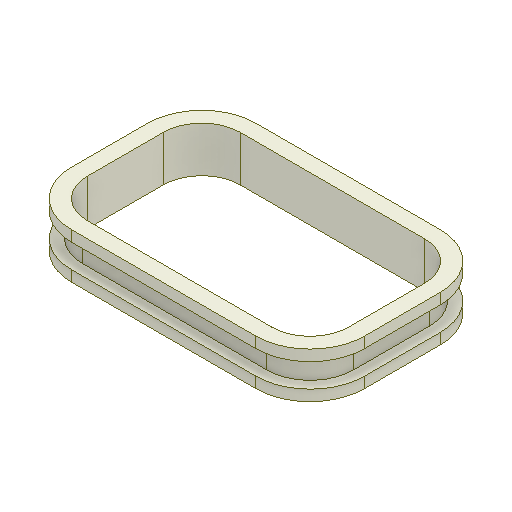
# Autodesk Inventor part: 3DP_TPU_Cable_Feed_Through_25mm
Saved by Autodesk Inventor 2026.1 (Build 301233000, 233)
## iProperties
Created: 2017-07-28
Part Number: 3DP_TPU_Cable_Feed_Through_25mm
Material: Ogólny
Document SubType Name: Modeling
Designer: Andrzej
Density: 1 g/cm^3
Appearance: Smooth - Ivory
Author: Andrzej
Autodesk Inventor part; units mm, degrees
ref_plane "YZ Plane" through (0, 0, 0) normal (1, 0, 0) x (0, 1, 0)
ref_plane "XZ Plane" through (0, 0, 0) normal (0, 1, 0) x (-1, 0, 0)
ref_plane "XY Plane" through (0, 0, 0) normal (0, 0, 1) x (1, 0, 0)
sketch "Szkic1" plane through (0, 0, 0) normal (0, 0, 1) x (1, 0, 0)
  line L0 (-2.3024, 6.9387) -> (14.6976, 6.9387)
  line L1 (18.6976, 2.9387) -> (18.6976, -4.0613)
  line L2 (14.6976, -8.0613) -> (-2.3024, -8.0613)
  line L3 (-6.3024, -4.0613) -> (-6.3024, 2.9387)
  arc A0 (-2.3024, 6.9387) -> (-6.3024, 2.9387) centre (-2.3024, 2.9387) ccw
  arc A1 (18.6976, 2.9387) -> (14.6976, 6.9387) centre (14.6976, 2.9387) ccw
  arc A2 (14.6976, -8.0613) -> (18.6976, -4.0613) centre (14.6976, -4.0613) ccw
  arc A3 (-6.3024, -4.0613) -> (-2.3024, -8.0613) centre (-2.3024, -4.0613) ccw
  line L4 (14.6976, 6.4887) -> (-2.3024, 6.4887)
  arc A4 (-2.3024, 6.4887) -> (-5.8524, 2.9387) centre (-2.3024, 2.9387) ccw
  line L5 (-5.8524, 2.9387) -> (-5.8524, -4.0613)
  arc A5 (-5.8524, -4.0613) -> (-2.3024, -7.6113) centre (-2.3024, -4.0613) ccw
  line L6 (-2.3024, -7.6113) -> (14.6976, -7.6113)
  arc A6 (14.6976, -7.6113) -> (18.2476, -4.0613) centre (14.6976, -4.0613) ccw
  line L7 (18.2476, -4.0613) -> (18.2476, 2.9387)
  arc A7 (18.2476, 2.9387) -> (14.6976, 6.4887) centre (14.6976, 2.9387) ccw
  point P0 (0, 0)
  point P1 (18.6976, -8.0613)
  point P2 (18.6976, 6.9387)
  point P3 (-6.3024, -8.0613)
  dimension "d0" = 25
  dimension "d1" = 15
  dimension "d2" = 4
  dimension "d3" = 0.45
  constraints: 16 end point, 16 point on circle, 8 centre point, 8 tangent, 6 point on line, 4 parallel, 3 equal radius, 2 perpendicular, 1 horizontal, 7 other
  measures "d0" distance of point (18.698, -8.061) point (-6.302, -8.061)
  measures "d1" distance of point (18.698, 6.939) point (18.698, -8.061)
  measures "d2" radius of A0
  measures "d3" distance between parallel lines of L0 L4
extrude "Wyciągnięcie proste1" add sketch "Szkic1" along normal blind 2.2
sketch "Szkic2" plane through (0, 0, 2.2) normal (0, 0, 1) x (1, 0, 0)
  arc A0 (18.2476, 2.9387) -> (14.6976, 6.4887) centre (14.6976, 2.9387) ccw projected
  line L0 (18.2476, 2.9387) -> (18.2476, -4.0613) projected
  arc A1 (14.6976, -7.6113) -> (18.2476, -4.0613) centre (14.6976, -4.0613) ccw projected
  line L1 (14.6976, -7.6113) -> (-2.3024, -7.6113) projected
  arc A2 (-5.8524, -4.0613) -> (-2.3024, -7.6113) centre (-2.3024, -4.0613) ccw projected
  line L2 (-5.8524, -4.0613) -> (-5.8524, 2.9387) projected
  arc A3 (-2.3024, 6.4887) -> (-5.8524, 2.9387) centre (-2.3024, 2.9387) ccw projected
  line L3 (-2.3024, 6.4887) -> (14.6976, 6.4887) projected
  line L4 (-6.3024, 2.9387) -> (-6.3024, -4.0613) projected
  arc A4 (-6.3024, -4.0613) -> (-2.3024, -8.0613) centre (-2.3024, -4.0613) ccw projected
  line L5 (-2.3024, -8.0613) -> (14.6976, -8.0613) projected
  arc A5 (14.6976, -8.0613) -> (18.6976, -4.0613) centre (14.6976, -4.0613) ccw projected
  line L6 (18.6976, -4.0613) -> (18.6976, 2.9387) projected
  arc A6 (18.6976, 2.9387) -> (14.6976, 6.9387) centre (14.6976, 2.9387) ccw projected
  line L7 (14.6976, 6.9387) -> (-2.3024, 6.9387) projected
  arc A7 (-2.3024, 6.9387) -> (-6.3024, 2.9387) centre (-2.3024, 2.9387) ccw projected
  line L8 (-7.3024, 2.9387) -> (-7.3024, -4.0613)
  arc A8 (-7.3024, -4.0613) -> (-2.3024, -9.0613) centre (-2.3024, -4.0613) ccw
  line L9 (-2.3024, -9.0613) -> (14.6976, -9.0613)
  arc A9 (14.6976, -9.0613) -> (19.6976, -4.0613) centre (14.6976, -4.0613) ccw
  line L10 (19.6976, -4.0613) -> (19.6976, 2.9387)
  arc A10 (19.6976, 2.9387) -> (14.6976, 7.9387) centre (14.6976, 2.9387) ccw
  line L11 (14.6976, 7.9387) -> (-2.3024, 7.9387)
  arc A11 (-2.3024, 7.9387) -> (-7.3024, 2.9387) centre (-2.3024, 2.9387) ccw
  point P0 (0, 0)
  dimension "d6" = 1
  constraints: 8 end point, 8 point on circle, 4 centre point, 7 other
  measures "d6" radial gap between concentric circles of A7 A11
extrude "Wyciągnięcie proste2" add sketch "Szkic2" along normal blind 1 contours A7 L7 A6 L6 A5 L5 A4 L4 | A11 L11 A10 L10 A9 L9 A8 L8
sketch "Szkic3" plane through (0, 0, 0) normal (0, 0, -1) x (-1, 0, 0)
  line L0 (7.3024, 2.9387) -> (7.3024, -4.0613) projected
  arc A0 (7.3024, 2.9387) -> (2.3024, 7.9387) centre (2.3024, 2.9387) ccw projected
  line L1 (-14.6976, 7.9387) -> (2.3024, 7.9387) projected
  arc A1 (-14.6976, 7.9387) -> (-19.6976, 2.9387) centre (-14.6976, 2.9387) ccw projected
  line L2 (-19.6976, -4.0613) -> (-19.6976, 2.9387) projected
  arc A2 (-19.6976, -4.0613) -> (-14.6976, -9.0613) centre (-14.6976, -4.0613) ccw projected
  line L3 (2.3024, -9.0613) -> (-14.6976, -9.0613) projected
  arc A3 (2.3024, -9.0613) -> (7.3024, -4.0613) centre (2.3024, -4.0613) ccw projected
  arc A4 (6.3024, 2.9387) -> (2.3024, 6.9387) centre (2.3024, 2.9387) ccw projected
  line L4 (6.3024, 2.9387) -> (6.3024, -4.0613) projected
  arc A5 (2.3024, -8.0613) -> (6.3024, -4.0613) centre (2.3024, -4.0613) ccw projected
  line L5 (2.3024, -8.0613) -> (-14.6976, -8.0613) projected
  arc A6 (-18.6976, -4.0613) -> (-14.6976, -8.0613) centre (-14.6976, -4.0613) ccw projected
  line L6 (-18.6976, -4.0613) -> (-18.6976, 2.9387) projected
  arc A7 (-14.6976, 6.9387) -> (-18.6976, 2.9387) centre (-14.6976, 2.9387) ccw projected
  line L7 (-14.6976, 6.9387) -> (2.3024, 6.9387) projected
  arc A8 (-14.6976, 6.4887) -> (-18.2476, 2.9387) centre (-14.6976, 2.9387) ccw projected
  line L8 (-14.6976, 6.4887) -> (2.3024, 6.4887) projected
  arc A9 (5.8524, 2.9387) -> (2.3024, 6.4887) centre (2.3024, 2.9387) ccw projected
  line L9 (5.8524, 2.9387) -> (5.8524, -4.0613) projected
  arc A10 (2.3024, -7.6113) -> (5.8524, -4.0613) centre (2.3024, -4.0613) ccw projected
  line L10 (2.3024, -7.6113) -> (-14.6976, -7.6113) projected
  arc A11 (-18.2476, -4.0613) -> (-14.6976, -7.6113) centre (-14.6976, -4.0613) ccw projected
  line L11 (-18.2476, -4.0613) -> (-18.2476, 2.9387) projected
  line L12 (6.3024, 2.9387) -> (6.3024, -4.0613) projected
  arc A12 (6.3024, 2.9387) -> (2.3024, 6.9387) centre (2.3024, 2.9387) ccw projected
  line L13 (-14.6976, 6.9387) -> (2.3024, 6.9387) projected
  arc A13 (-14.6976, 6.9387) -> (-18.6976, 2.9387) centre (-14.6976, 2.9387) ccw projected
  line L14 (-18.6976, -4.0613) -> (-18.6976, 2.9387) projected
  arc A14 (-18.6976, -4.0613) -> (-14.6976, -8.0613) centre (-14.6976, -4.0613) ccw projected
  line L15 (2.3024, -8.0613) -> (-14.6976, -8.0613) projected
  arc A15 (2.3024, -8.0613) -> (6.3024, -4.0613) centre (2.3024, -4.0613) ccw projected
  point P0 (0, 0)
extrude "Wyciągnięcie proste3" add sketch "Szkic3" along normal blind 1 contours L0 A3 L3 A2 L2 A1 L1 A0 | L4 A5 L5 A6 L6 A7 L7 A4
